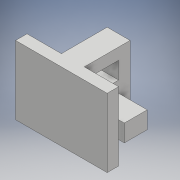
# Autodesk Inventor part: P3-8
Saved by Autodesk Inventor 2017 (Build 210142000, 142)
## iProperties
Created: 2017-02-12
Part Number: P3-8
Material: Generic
Document SubType Name: Modeling
Designer: Schaffel
Density: 1 g/cm^3
Appearance: Default
Author: Schaffel
Autodesk Inventor part; units mm, degrees
ref_plane "YZ Plane" through (0, 0, 0) normal (1, 0, 0) x (0, 1, 0)
ref_plane "XZ Plane" through (0, 0, 0) normal (0, 1, 0) x (-1, 0, 0)
ref_plane "XY Plane" through (0, 0, 0) normal (0, 0, 1) x (1, 0, 0)
sketch "Sketch1" plane through (0, 0, 0) normal (0, 0, 1) x (1, 0, 0)
  line L0 (0, 0) -> (80, 0)
  line L1 (80, 0) -> (80, 10)
  line L2 (80, 10) -> (50, 10)
  line L3 (50, 10) -> (50, 50)
  line L4 (50, 50) -> (30, 50)
  line L5 (30, 50) -> (30, 10)
  line L6 (30, 10) -> (0, 10)
  line L7 (0, 10) -> (0, 0)
  dimension "d0" = 80
  dimension "d1" = 10
  dimension "d2" = 40
  constraints: 16 end point, 6 perpendicular, 2 point on line, 1 horizontal
  measures "d0" distance of L0.start L0.end
  measures "d1" distance of L0.end L1.end
  measures "d2" distance of L2.end L3.end
extrude "Extrusion1" add sketch "Sketch1" along normal blind 60
sketch "Sketch2" plane through (50, 10, 0) normal (1, 0, 0) x (0, 0, -1)
  line L0 (-10, 10) -> (-25, 10)
  line L1 (-25, 10) -> (-25, 30)
  line L2 (-25, 30) -> (-10, 30)
  line L3 (-10, 30) -> (-10, 10)
  line L4 (-50, 30) -> (-50, 10)
  line L5 (-50, 10) -> (-35, 10)
  line L6 (-35, 10) -> (-35, 30)
  line L7 (-35, 30) -> (-50, 30)
  point P0 (0, -10)
  constraints: 16 end point, 6 perpendicular, 1 horizontal, 1 vertical
extrude "Extrusion2" add sketch "Sketch2" along normal blind 25 contours L0 L1 L2 L3
sketch "Sketch3" plane through (50, 10, 0) normal (1, 0, 0) x (0, 0, -1)
  line L0 (-35, 30) -> (-35, 10)
  line L1 (-35, 10) -> (-50, 10)
  line L2 (-50, 10) -> (-50, 30)
  line L3 (-60, 40) -> (-60, 0) projected
  line L4 (-50, 30) -> (-35, 30)
  point P0 (0, -10)
  constraints: 8 end point, 2 perpendicular, 1 parallel, 1 vertical
extrude "Extrusion3" cut sketch "Sketch3" against normal blind 20
body "Solid1"
